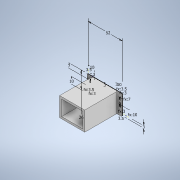
# Autodesk Inventor part: battery
Saved by Autodesk Inventor 2020 (Build 240168000, 168)
## iProperties
Created: 2022-09-29
Part Number: battery
Material: 일반
Document SubType Name: Modeling
Designer: taewo
Density: 1 g/cm^3
Appearance: 기본값
Author: taewo
Autodesk Inventor part; units mm, degrees
ref_plane "YZ Plane" through (0, 0, 0) normal (1, 0, 0) x (0, 1, 0)
ref_plane "XZ Plane" through (0, 0, 0) normal (0, 1, 0) x (-1, 0, 0)
ref_plane "XY Plane" through (0, 0, 0) normal (0, 0, 1) x (1, 0, 0)
sketch "스케치1" plane through (0, 0, 0) normal (0, 0, 1) x (1, 0, 0)
  line L0 (-10.4, 0) -> (62.4, 0) construction
  line L1 (0, -8.8) -> (0, 31.8) construction
  line L2 (0, 26) -> (52, 26)
  line L3 (52, 26) -> (52, 0)
  line L4 (52, 0) -> (0, 0)
  line L5 (0, 0) -> (0, 26)
  circle A0 centre (3.5, 19) radius 1.5
  circle A1 centre (3.5, 10) radius 1.5
  circle A2 centre (48.5, 19) radius 1.5
  circle A3 centre (48.5, 10) radius 1.5
  line L6 (10, 23) -> (42, 23)
  line L7 (42, 23) -> (42, 0)
  line L8 (42, 0) -> (10, 0)
  line L9 (10, 0) -> (10, 23)
  line L10 (0, 0) -> (52, 0)
  line L11 (52, 0) -> (52, -3)
  line L12 (52, -3) -> (0, -3)
  line L13 (0, -3) -> (0, 0)
  line L14 (7, 23) -> (10, 23)
  line L15 (10, 23) -> (10, 0)
  line L16 (10, 0) -> (7, 0)
  line L17 (7, 0) -> (7, 23)
  line L18 (42, 23) -> (45, 23)
  line L19 (45, 23) -> (45, 0)
  line L20 (45, 0) -> (42, 0)
  line L21 (42, 0) -> (42, 23)
  line L22 (0, 23) -> (7, 23)
  line L23 (45, 23) -> (52, 23)
  line L24 (7, 26) -> (7, 22.7671)
  line L25 (45, 26) -> (45, 23)
  line L26 (7, 0) -> (7, -3)
  line L27 (45, 0) -> (45, -3)
  point P0 (52, 0)
  dimension "d0" = 26
  dimension "d1" = 52
  dimension "d2" = 3
  dimension "d3" = 3
  dimension "d4" = 3
  dimension "d5" = 3
  dimension "d6" = 3.5
  dimension "d7" = 3.5
  dimension "d8" = 3.5
  dimension "d10" = 7
  dimension "d11" = 7
  dimension "d12" = 10
  dimension "d13" = 10
  dimension "d14" = 3
  dimension "d15" = 10
  dimension "d16" = 10
  dimension "d17" = 3
  dimension "d18" = 3
  dimension "d19" = 3
  dimension "d20" = 3.5
  constraints: 52 end point, 10 parallel, 10 point on line, 8 perpendicular, 5 horizontal, 4 centre point, 3 collinear
  measures "d0" distance of L4.end L2.start
  measures "d1" distance of L2.start L2.end
  measures "d2" diameter of A0
  measures "d3" diameter of A1
  measures "d4" diameter of A2
  measures "d5" diameter of A3
  measures "d6" distance from line of L5 A0.centre
  measures "d7" distance from line of L1 A1.centre
  measures "d8" distance from line of L3 A2.centre
  measures "d10" distance from line of L2 A0.centre
  measures "d11" distance from line of L2 A2.centre
  measures "d12" distance from line of L0 A1.centre
  measures "d13" distance from line of L4 A3.centre
  measures "d14" distance between parallel lines of L2 L6
  measures "d15" distance between parallel lines of L5 L9
  measures "d16" distance between parallel lines of L3 L7
  measures "d17" distance of L10.end L11.end
  measures "d18" distance of L14.start L14.end
  measures "d19" distance of L6.end L18.end
  measures "d20" distance from line of L3 A3.centre
extrude "돌출1" add sketch "스케치1" along normal blind 50 contours L2 L25 L18 L6 L14 L24 | L14 L9 L4 L17 | L19 L4 L7 L18 | L4 L27 L12 L26
extrude "돌출2" add sketch "스케치1" along normal blind 1.5 contours L2 L24 L22 L5 | L22 L17 L4 L5 | L2 L3 L23 L25 | L4 L26 L12 L13 | L23 L3 L4 L19 | L4 L11 L12 L27
equation "\"d3\" = d2"
equation "\"d4\" = d2"
equation "\"d5\" = d2"
equation "\"d7\" = d6"
equation "\"d8\" = d6"
equation "\"d11\" = d10"
equation "\"d13\" = d12"
